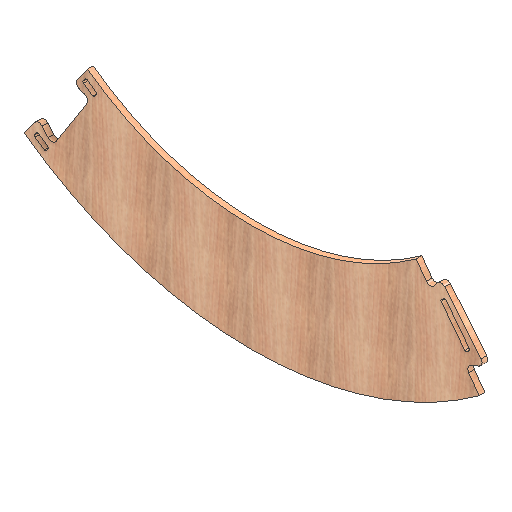
# Autodesk Inventor part: Platform E2
Saved by Autodesk Inventor 2021 (Build 250183000, 183)
## iProperties
Created: 2020-05-09
Part Number: Platform E2
Material: Wood (Birch)
Document SubType Name: Modeling
Designer: Dan Wikman
Density: 0.55 g/cm^3
Appearance: Birch - Natural Polished
Mass: 4367.89 g
Surface Area: 9554.9 cm^2
Volume: 7941.62 cm^3
Autodesk Inventor part; units mm, degrees
ref_plane "YZ Plane" through (0, 0, 0) normal (1, 0, 0) x (0, 1, 0)
ref_plane "XZ Plane" through (0, 0, 0) normal (0, 1, 0) x (-1, 0, 0)
ref_plane "XY Plane" through (0, 0, 0) normal (0, 0, 1) x (1, 0, 0)
sketch "CONTOURS" plane through (0, 0, 0) normal (0, 0, 1) x (1, 0, 0)
  arc A0 (122.9585, 280.6191) -> (147.7621, 282.3295) centre (134.7234, 290.7105) ccw
  line L0 (147.7621, 282.3295) -> (245.0646, 433.7067)
  arc A1 (245.0646, 433.7067) -> (237.169, 456.7096) centre (232.0259, 442.0877) ccw
  line L1 (237.169, 456.7096) -> (221.2353, 462.314)
  arc A2 (214.3157, 484.5154) -> (221.2353, 462.314) centre (226.0465, 475.9926) ccw
  line L2 (214.3157, 484.5154) -> (246.7015, 529.0906)
  arc A3 (246.7015, 529.0906) -> (1281.107, 529.0906) centre (763.9042, 1241.8098) ccw
  line L3 (1281.107, 529.0906) -> (1313.4927, 484.5154)
  arc A4 (1313.4927, 484.5154) -> (1338.3495, 484.2164) centre (1326.0325, 493.6261) ccw
  line L4 (1338.3495, 484.2164) -> (1348.6034, 497.6384)
  arc A5 (1371.3515, 498.0135) -> (1348.6034, 497.6384) centre (1360.1257, 488.8357) ccw
  line L5 (1371.3515, 498.0135) -> (1485.2517, 358.6952)
  arc A6 (1479.6031, 336.133) -> (1485.2517, 358.6952) centre (1474.0258, 349.5174) ccw
  line L6 (1479.6031, 336.133) -> (1452.9579, 325.03)
  arc A7 (1452.9579, 325.03) -> (1446.3801, 301.6117) centre (1458.9198, 310.7224) ccw
  line L7 (1446.3801, 301.6117) -> (1479.7785, 255.6428)
  arc A8 (48.0301, 255.6429) -> (1479.7785, 255.6428) centre (763.9044, 1242.1407) ccw
  line L8 (48.0301, 255.6429) -> (81.4284, 301.6117)
  arc A9 (104.1651, 302.5292) -> (81.4284, 301.6117) centre (93.1592, 293.0889) ccw
  line L9 (104.1651, 302.5292) -> (122.9585, 280.6191)
  constraints: 20 end point, 20 point on circle, 10 centre point
sketch "HOLES" plane through (0, 0, 0) normal (0, 0, 1) x (1, 0, 0)
  arc A0 (123.1485, 251.2322) -> (122.1121, 256.7934) centre (119.8497, 253.4946) ccw
  line L0 (122.1121, 256.7934) -> (92.4235, 277.1548)
  arc A1 (92.4235, 277.1548) -> (86.8624, 276.1184) centre (90.1611, 273.856) ccw
  line L1 (86.8624, 276.1184) -> (80.6409, 267.0469)
  arc A2 (80.6409, 267.0469) -> (81.6772, 261.4858) centre (83.9396, 264.7845) ccw
  line L2 (116.9269, 242.1607) -> (123.1485, 251.2322)
  arc A3 (111.3658, 241.1244) -> (116.9269, 242.1607) centre (113.6282, 244.4231) ccw
  line L3 (264.0494, 464.2922) -> (234.3609, 484.6537)
  arc A4 (233.3245, 490.2148) -> (234.3609, 484.6537) centre (236.6232, 487.9524) ccw
  line L4 (233.3245, 490.2148) -> (239.546, 499.2863)
  arc A5 (245.1072, 500.3226) -> (239.546, 499.2863) centre (242.8448, 497.0239) ccw
  line L5 (245.1072, 500.3226) -> (274.7957, 479.9612)
  arc A6 (275.8321, 474.4001) -> (274.7957, 479.9612) centre (272.5334, 476.6625) ccw
  line L6 (275.8321, 474.4001) -> (269.6106, 465.3286)
  arc A7 (264.0494, 464.2922) -> (269.6106, 465.3286) centre (266.3118, 467.591) ccw
  line L7 (1443.1181, 358.0576) -> (1448.6625, 362.3307)
  arc A8 (1448.6625, 362.3307) -> (1449.389, 367.9407) centre (1446.2207, 365.4989) ccw
  line L8 (1449.389, 367.9407) -> (1374.9151, 464.5722)
  arc A9 (1374.9151, 464.5722) -> (1369.3051, 465.2986) centre (1371.7469, 462.1304) ccw
  line L9 (1369.3051, 465.2986) -> (1360.5924, 458.5838)
  arc A10 (1360.5924, 458.5838) -> (1359.866, 452.9738) centre (1363.0342, 455.4155) ccw
  line L10 (1359.866, 452.9738) -> (1434.3398, 356.3423)
  arc A11 (1434.3398, 356.3423) -> (1439.9498, 355.6158) centre (1437.5081, 358.7841) ccw
  line L11 (1439.9498, 355.6158) -> (1443.1181, 358.0576)
  line L12 (81.6772, 261.4858) -> (111.3658, 241.1244)
  constraints: 26 end point, 24 point on circle, 12 centre point
sketch "LETTERS" plane through (0, 0, 0) normal (0, 0, 1) x (1, 0, 0)
  line L0 (274.8207, 322.605) -> (262.022, 329.8103)
  line L1 (262.022, 329.8103) -> (252.3047, 312.5498)
  line L2 (252.3047, 312.5498) -> (265.1034, 305.3445)
  constraints: 6 end point
extrude "Extrusion1" add sketch "CONTOURS" along normal blind 18
extrude "Extrusion2" cut sketch "HOLES" along normal blind 18
body "Solid1"
